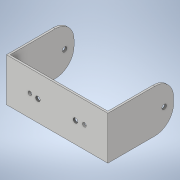
# Autodesk Inventor part: 20220523_servo_iron.0001
Saved by Autodesk Inventor 2020 (Build 240168000, 168)
## iProperties
Created: 2021-06-29
Part Number: 20220523_servo_iron.0001
Material: 一般
Document SubType Name: Modeling
Designer: fmasa
Density: 1 g/cm^3
Appearance: 既定
Author: fmasa
Autodesk Inventor part; units mm, degrees
ref_plane "YZ Plane" through (0, 0, 0) normal (1, 0, 0) x (0, 1, 0)
ref_plane "XZ Plane" through (0, 0, 0) normal (0, 1, 0) x (-1, 0, 0)
ref_plane "XY Plane" through (0, 0, 0) normal (0, 0, 1) x (1, 0, 0)
sketch "スケッチ1" plane through (0, 0, 0) normal (0, 0, 1) x (1, 0, 0)
  line L0 (0, 0) -> (54, 0)
  line L1 (54, 0) -> (54, 23)
  line L2 (54, 23) -> (0, 23)
  line L3 (0, 23) -> (0, 0)
  circle A0 centre (27, 11.5) radius 14.5 construction
  line L4 (-4.1299, 11.5) -> (79.808, 11.5) construction
  line L5 (27, 36.9119) -> (27, -8.8804) construction
  circle A1 centre (12.5, 11.5) radius 1
  circle A2 centre (41.5, 11.5) radius 1
  dimension "d0" = 54
  dimension "d1" = 23
  dimension "d2" = 29
  dimension "d3" = 2
  dimension "d4" = 2
  constraints: 12 end point, 3 centre point, 2 horizontal, 2 parallel, 2 point on circle, 1 perpendicular, 1 point on line, 1 vertical
  measures "d0" distance of L2.end L1.end
  measures "d1" distance of L1.end L0.end
  measures "d2" diameter of A0
  measures "d3" diameter of A1
  measures "d4" diameter of A2
extrude "押し出し1" add sketch "スケッチ1" along normal blind 1
sketch "スケッチ2" plane through (0, 0, 0) normal (0, 0, -1) x (-1, 0, 0)
  line L0 (0, 0) -> (-54, 0) projected
  line L1 (-54, 23) -> (0, 23) projected
  line L2 (0, 0) -> (-1, 0)
  line L3 (-1, 0) -> (-1, 23)
  line L4 (-1, 23) -> (0, 23)
  line L5 (0, 23) -> (0, 0)
  line L6 (-54, 0) -> (-54, 23) projected
  line L7 (-54, 0) -> (-53, 0)
  line L8 (-53, 0) -> (-53, 23)
  line L9 (-53, 23) -> (-54, 23)
  line L10 (-54, 23) -> (-54, 0)
  dimension "d7" = 1
  dimension "d8" = 1
  constraints: 16 end point, 4 parallel, 2 horizontal, 2 perpendicular, 2 point on line
  measures "d7" distance of L3.end L4.end
  measures "d8" distance of L9.end L8.end
extrude "押し出し2" add sketch "スケッチ2" along normal blind 34 contours L0 L3 L1 L5 | L0 L6 L1 L8
fillet "フィレット1" radius 10 4 edges at (53.5, 23, -34) (53.5, 0, -34) (0.5, 0, -34) (0.5, 23, -34)
sketch "スケッチ4" plane through (0, 0, 1) normal (-1, 0, 0) x (0, 0, 1)
  line L0 (0, 23) -> (0, 0) projected
  line L1 (0, 0) -> (-25, 0) projected
  point P0 (-1, 0)
  point P1 (-30, 11)
  dimension "d21" = 30
  dimension "d22" = 11
  measures "d21" distance from line of point (-30, 11) L0
  measures "d22" distance from line of point (-30, 11) L1
hole "穴2" at (0, 11, -29) direction (1, 0, 0) diameter 2.459 depth 8.8 tip angle 118 thread size "M3x0.5" class "6H" standard "ANSI Metric M Profile"
sketch "スケッチ5" plane through (54, 0, 1) normal (1, 0, 0) x (0, 0, -1)
  line L0 (0, 0) -> (0, 23) projected
  line L1 (25, 0) -> (0, 0) projected
  point P0 (1, 0)
  point P1 (30, 11)
  dimension "d30" = 30
  dimension "d31" = 11
  measures "d30" distance from line of point (30, 11) L0
  measures "d31" distance from line of point (30, 11) L1
hole "穴3" at (54, 11, -29) direction (-1, 0, 0) diameter 2.459 depth 8.8 tip angle 118 thread size "M3x0.5" class "6H" standard "ANSI Metric M Profile"
sketch "スケッチ6" plane through (0, 0, 1) normal (0, 0, 1) x (1, 0, 0)
  line L0 (0, 23) -> (0, 0) projected
  point P0 (16.7596, 11.0453)
  point P1 (100, 11.0453)
  point P2 (36.7596, 11.0453)
  dimension "d39" = 20
  dimension "d40" = 100
  measures "d39" distance of point (36.76, 11.045) point (16.76, 11.045)
  measures "d40" distance from line of L0 point (100, 11.045)
hole "穴4" at (16.7596, 11.0453, 1) at (100, 11.0453, 1) at (36.7596, 11.0453, 1) direction (0, 0, -1) diameter 2.459 depth 8.8 tip angle 118 thread size "M3x0.5" class "6H" standard "ANSI Metric M Profile"
